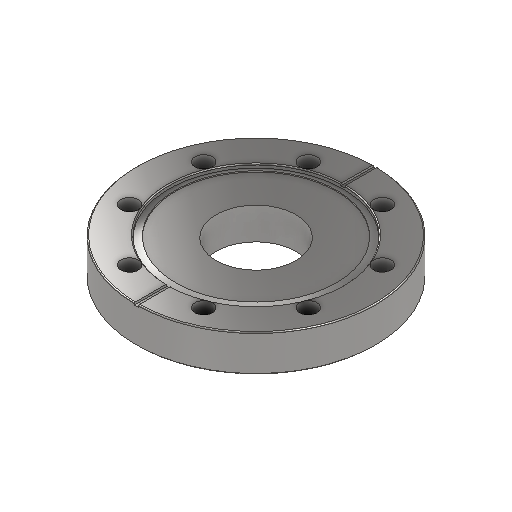
# Autodesk Inventor part: CF_114-70
Saved by Autodesk Inventor 2026.2 (Build 302298000, 298)
## iProperties
Created: 2026-03-22
Part Number: CF_114-70
Material: ステンレス鋼 440C
Document SubType Name: Modeling
Designer: zetsu
Density: 7.75 g/cm^3
Appearance: 半つや出し
Author: zetsu
Autodesk Inventor part; units mm, degrees
ref_plane "YZ Plane" through (0, 0, 0) normal (1, 0, 0) x (0, 1, 0)
ref_plane "XZ Plane" through (0, 0, 0) normal (0, 1, 0) x (-1, 0, 0)
ref_plane "XY Plane" through (0, 0, 0) normal (0, 0, 1) x (1, 0, 0)
sketch "スケッチ1" plane through (0, 0, 0) normal (0, 0, 1) x (1, 0, 0)
  line L0 (24.105, -0.1673) -> (57, -0.1673)
  line L1 (57, -0.1673) -> (57, 17.3327)
  line L2 (57, 17.3327) -> (41.531, 17.3327)
  line L3 (19, 16.5132) -> (19, 1.0007)
  line L4 (0, 0) -> (0, 34.98) construction
  line L5 (41.531, 17.3327) -> (41.531, 15.5077)
  line L6 (41.531, 15.5077) -> (38.331, 16.6727)
  line L7 (38.331, 16.6727) -> (38.331, 16.1647)
  line L8 (38.331, 16.1647) -> (19, 16.1647)
  line L9 (24.105, -0.1673) -> (24.105, 1.6577)
  line L10 (24.105, 1.6577) -> (20.905, 0.4927)
  line L11 (20.905, 0.4927) -> (20.905, 1.0007)
  line L12 (20.905, 1.0007) -> (19, 1.0007)
  dimension "d2" = 17.5
  dimension "d3" = 1.825
  dimension "d4" = 3.2
  dimension "d5" = 0.657
  dimension "d7" = 38
  dimension "d8" = 15.469
  dimension "d9" = 5.105
  dimension "d10" = 19
  dimension "d11" = 1.825
  dimension "d12" = 1.165
  dimension "d13" = 1.165
  dimension "d14" = 0.657
  dimension "d15" = 3.2
  constraints: 26 end point, 4 parallel, 4 perpendicular, 2 vertical, 1 horizontal, 1 point on line
  measures "d2" distance of L0.end L1.end
  measures "d3" distance of L2.end L5.end
  measures "d4" horizontal distance of L5.end L6.end
  measures "d5" vertical distance of L5.end L7.end
  measures "d7" horizontal distance of L1.end L3.start
  measures "d8" distance of L1.end L2.end
  measures "d9" horizontal distance of L0.start L3.end
  measures "d10" horizontal distance of L3.start L4.start
  measures "d11" distance of L0.start L9.end
  measures "d12" vertical distance of L5.end L6.end
  measures "d13" vertical distance of L9.end L10.end
  measures "d14" vertical distance of L9.end L11.end
  measures "d15" horizontal distance of L9.end L10.end
revolve "回転1" add sketch "スケッチ1" angle 360 about axis through (0, 0, 0) along (0, 1, 0)
sketch "スケッチ2" plane through (0, 17.3327, 0) normal (0, 1, 0) x (1, 0, 0)
  circle A0 centre (-42.6139, -17.6513) radius 4.2165
  circle A1 centre (-17.6513, -42.6139) radius 4.2165
  circle A2 centre (17.6513, -42.6139) radius 4.2165
  circle A3 centre (42.6139, -17.6513) radius 4.2165
  circle A4 centre (42.6139, 17.6513) radius 4.2165
  circle A5 centre (17.6513, 42.6139) radius 4.2165
  circle A6 centre (-17.6513, 42.6139) radius 4.2165
  circle A7 centre (-42.6139, 17.6513) radius 4.2165
  point P0 (0, 0)
  dimension "d17" = 8.433
  dimension "d18" = 46.125
  dimension "d21" = 360
  constraints: 8 centre point, 17 other
  measures "d17" diameter of A0
  measures "d18" distance of point (0, 0) A0.centre
extrude "押し出し1" cut sketch "スケッチ2" against normal through all
sketch "スケッチ3" plane through (0, -0.1673, 0) normal (0, -1, 0) x (1, 0, 0)
  circle A0 centre (0, 29.369) radius 2.705
  circle A1 centre (-25.4343, 14.6845) radius 2.705
  circle A2 centre (-25.4343, -14.6845) radius 2.705
  circle A3 centre (0, -29.369) radius 2.705
  circle A4 centre (25.4343, -14.6845) radius 2.705
  circle A5 centre (25.4343, 14.6845) radius 2.705
  point P0 (0, 0)
  dimension "d25" = 5.41
  dimension "d26" = 29.369
  dimension "d29" = 360
  constraints: 6 centre point, 13 other
  measures "d25" diameter of A0
  measures "d26" distance of point (0, 0) A0.centre
extrude "押し出し2" cut sketch "スケッチ3" against normal blind 10
fillet "フィレット1" radius 0.5 4 edges at (-57, 17.3327, 0) (-57, -0.1673, 0) (-41.531, 17.3327, 0) (-24.105, -0.1673, 0)
sketch "スケッチ4" plane through (0, 17.3327, 0) normal (0, 1, 0) x (1, 0, 0)
  line L0 (-1, 58.1899) -> (1, 58.1899)
  line L1 (1, 58.1899) -> (1, 40.9721)
  line L2 (1, 40.9721) -> (-1, 40.9721)
  line L3 (-1, 40.9721) -> (-1, 58.1899)
  line L4 (0, 0) -> (0, 179.4952) construction
  line L5 (-1, -40.4733) -> (1, -40.4733)
  line L6 (1, -40.4733) -> (1, -60.385)
  line L7 (1, -60.385) -> (-1, -60.385)
  line L8 (-1, -60.385) -> (-1, -40.4733)
  dimension "d34" = 2
  dimension "d35" = 2
  constraints: 18 end point, 4 parallel, 2 horizontal, 2 perpendicular, 1 vertical, 2 other
  measures "d34" distance of L0.start L0.end
  measures "d35" distance of L6.end L7.end
extrude "押し出し3" cut sketch "スケッチ4" against normal blind 1
